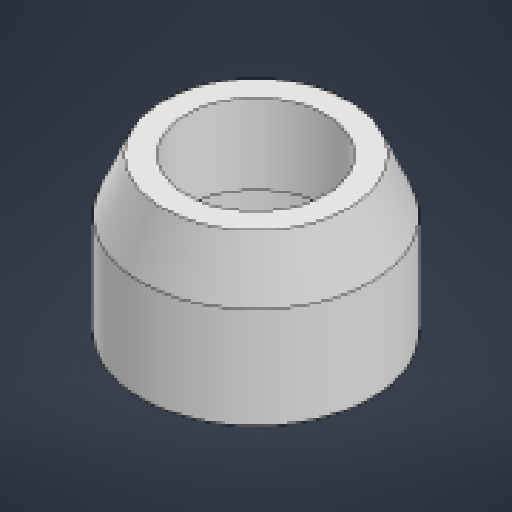
# Autodesk Inventor part: LimitedView_Parts
Saved by Autodesk Inventor 2024.2 (Build 282272000, 272)
## iProperties
Created: 2024-01-10
Part Number: LimitedView_Parts
Material: 一般
Document SubType Name: Modeling
Designer: Hanaoka
Density: 1 g/cm^3
Appearance: 既定
Author: Hanaoka
Autodesk Inventor part; units mm, degrees
ref_plane "YZ Plane" through (0, 0, 0) normal (1, 0, 0) x (0, 1, 0)
ref_plane "XZ Plane" through (0, 0, 0) normal (0, 1, 0) x (-1, 0, 0)
ref_plane "XY Plane" through (0, 0, 0) normal (0, 0, 1) x (1, 0, 0)
ref_plane "作業平面1" through (0, 0, 0) normal (0, 0, 1) x (1, 0, 0)
sketch "スケッチ1" plane through (0, 0, 0) normal (0, 0, 1) x (1, 0, 0)
  line L0 (14.5, 10.3) -> (0.5, 10.3) projected
  line L1 (-0.25, 6.3) -> (15.25, 6.3) projected
  line L2 (19.4, 0) -> (17.5, 0) projected
  line L3 (-2.5, 0) -> (-4.4, 0) projected
  line L4 (15, -8) -> (0, -8) projected
  line L5 (7.5, 10.3) -> (7.5, -8)
  line L6 (-16.5, -5.5) -> (31.5, -5.5) projected
  line L7 (20.9, 4) -> (20.9, -5.5)
  line L8 (22.4, 7.5) -> (22.4, -5.5)
  line L9 (16.5, 14.3) -> (19.5, 14.3)
  line L10 (19.5, 14.3) -> (22.4, 7.5)
  line L11 (20.9, 4) -> (16.5, 4)
  line L12 (16.5, 4) -> (16.5, 14.3)
  line L13 (20.9, -5.5) -> (22.4, -5.5)
  point P0 (0, 0)
  dimension "d2" = 1.5
  dimension "d4" = 3
  dimension "d5" = 1.5
  dimension "d6" = 13
  dimension "d7" = 1.25
  dimension "d8" = 4
  dimension "d9" = 4
  constraints: 16 end point, 2 horizontal, 2 midpoint, 2 perpendicular, 2 point on line, 1 collinear, 1 vertical
  measures "d2" distance from line of L7 L2.start
  measures "d4" distance of L9.start L9.end
  measures "d5" distance between parallel lines of L7 L8
  measures "d6" distance of L8.start L8.end
  measures "d7" horizontal distance of L1.end L11.end
  measures "d8" distance between parallel lines of L2 L11
  measures "d9" vertical distance of L9.start L0.start
revolve "回転1" add sketch "スケッチ1" angle 360 about axis through (7.5, 10.3, 0) along (0, -1, 0)
